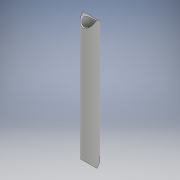
# Autodesk Inventor part: 縦のパイプ
Saved by Autodesk Inventor 2018 (Build 220112000, 112)
## iProperties
Created: 2017-09-10
Part Number: 縦のパイプ
Material: 一般
Document SubType Name: Modeling
Designer: Kenta
Density: 1 g/cm^3
Appearance: 既定
Author: Kenta
Autodesk Inventor part; units mm, degrees
ref_plane "YZ Plane" through (0, 0, 0) normal (1, 0, 0) x (0, 1, 0)
ref_plane "XY Plane" through (0, 0, 0) normal (0, 0, 1) x (1, 0, 0)
sketch "スケッチ1" plane through (0, 0, 0) normal (0, 0, 1) x (1, 0, 0)
  circle A0 centre (0, 0) radius 13.6
  dimension "d0" = 27.2
  constraints: 1 centre point, 1 coincident
  measures "d0" diameter of A0
extrude "押し出し1" add sketch "スケッチ1" against normal blind 250
sketch "スケッチ3" plane through (0, 0, 0) normal (0, 0, 1) x (1, 0, 0)
  circle A0 centre (0, 0) radius 13.6 projected
  constraints: 1 coincident
hole "穴1" at (0, 0, 0) direction (0, 0, -1) diameter 22.6 end through all
ref_plane "作業平面1" through (0, 0, 0) normal (0, 1, 0) x (-1, 0, 0)
sketch "スケッチ4" plane through (0, 0, 0) normal (0, 1, 0) x (-1, 0, 0)
  line L0 (-13.6, 0) -> (13.6, 0) projected
  arc A0 (-13.6, 0) -> (13.6, 0) centre (0, 0) ccw
  line L1 (13.6, 0) -> (-13.6, 0)
  constraints: 2 end point, 2 point on circle, 1 centre point, 1 coincident, 1 collinear
extrude "押し出し3" cut sketch "スケッチ4" along normal mid plane 27.2
sketch "スケッチ5" plane through (0, 0, 0) normal (0, 1, 0) x (-1, 0, 0)
  line L0 (-13.6, -250) -> (13.6, -250) projected
  arc A0 (13.6, -250) -> (-13.6, -250) centre (0, -250) ccw
  line L1 (-13.6, -250) -> (13.6, -250)
  point P0 (0, 0)
  constraints: 2 end point, 2 point on circle, 1 centre point, 1 horizontal
extrude "押し出し4" cut sketch "スケッチ5" along normal mid plane 27.2
